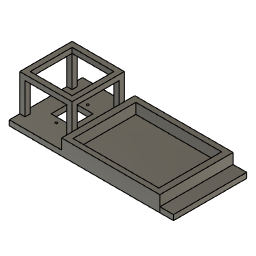
PDMS holder v6 (Autodesk Fusion 360 design; units mm, degrees)
Autodesk Fusion 360 part; units mm, degrees
sketch "Sketch1" plane through (0, 0, 0) normal (0, 0, 1) x (1, 0, 0)
  line L0 (12.5, -12.5) -> (-12.5, -12.5)
  line L1 (-12.5, -12.5) -> (-12.5, 12.5)
  line L2 (-12.5, 12.5) -> (12.5, 12.5)
  line L3 (12.5, 12.5) -> (12.5, -12.5)
  line L4 (12.5, -12.5) -> (-12.5, 12.5) construction
  line L5 (-12.5, -12.5) -> (12.5, 12.5) construction
  line L6 (10, -10) -> (-10, -10)
  line L7 (-10, -10) -> (-10, 10)
  line L8 (-10, 10) -> (10, 10)
  line L9 (10, 10) -> (10, -10)
  line L10 (10, -10) -> (-10, 10) construction
  line L11 (-10, -10) -> (10, 10) construction
  line L12 (5, -5) -> (-5, -5)
  line L13 (-5, -5) -> (-5, 5)
  line L14 (-5, 5) -> (5, 5)
  line L15 (5, 5) -> (5, -5)
  line L16 (5, -5) -> (-5, 5) construction
  line L17 (-5, -5) -> (5, 5) construction
  line L18 (12.5, 0) -> (12.5, 17.5)
  line L19 (12.5, 17.5) -> (59.5, 17.5)
  line L20 (59.5, 17.5) -> (59.5, -17.5)
  line L21 (59.5, -17.5) -> (12.5, -17.5)
  line L22 (12.5, -17.5) -> (12.5, 17.5)
  line L23 (12.5, 0) -> (36, 0)
  line L24 (56.5, -15) -> (15.5, -15)
  line L25 (15.5, -15) -> (15.5, 15)
  line L26 (15.5, 15) -> (56.5, 15)
  line L27 (56.5, 15) -> (56.5, -15)
  line L28 (56.5, -15) -> (15.5, 15) construction
  line L29 (15.5, -15) -> (56.5, 15) construction
  line L30 (12.5, -17.5) -> (-12.5, -17.5)
  line L31 (-12.5, -17.5) -> (-12.5, 17.5)
  line L32 (-12.5, 17.5) -> (12.5, 17.5)
  line L33 (12.5, 17.5) -> (12.5, -17.5)
  line L34 (0, 0) -> (0, 7.5)
  line L35 (0, 7.5) -> (0, -7.5)
  circle A0 centre (0, 7.5) radius 0.5
  circle A1 centre (0, -7.5) radius 0.5
  line L36 (59.5, 17.5) -> (66, 17.5)
  line L37 (66, 17.5) -> (66, -17.5)
  line L38 (66, -17.5) -> (59.5, -17.5)
  line L39 (59.5, -17.5) -> (59.5, 17.5)
  point P0 (36, 0)
  dimension "d1" = 25
  dimension "d2" = 25
  dimension "d3" = 20
  dimension "d4" = 20
  dimension "d19" = 10
  dimension "d20" = 10
  dimension "d25" = 17.5
  dimension "d26" = 47
  dimension "d27" = 35
  dimension "d28" = 23.5
  dimension "d29" = 41
  dimension "d30" = 30
  dimension "d33" = 25
  dimension "d34" = 35
  dimension "d35" = 7.5
  dimension "d36" = 15
  dimension "d37" = 1
  dimension "d38" = 1
  dimension "d39" = 6.5
  dimension "d40" = 35
  constraint horizontal L0
  constraint perpendicular L0 L1
  constraint parallel L0 L2
  constraint parallel L1 L3
  constraint coincident L4 L34.start
  constraint coincident L5 L34.start
  constraint coincident L34.start origin
  constraint horizontal L6
  constraint perpendicular L6 L7
  constraint parallel L6 L8
  constraint parallel L7 L9
  constraint coincident L10 L34.start
  constraint coincident L11 L34.start
  constraint horizontal L12
  constraint perpendicular L12 L13
  constraint parallel L12 L14
  constraint parallel L13 L15
  constraint coincident L16 L34.start
  constraint coincident L17 L34.start
  constraint midpoint L3 L18.start
  constraint perpendicular L2 L18
  constraint horizontal L19
  constraint vertical L20
  constraint horizontal L21
  constraint vertical L22
  constraint perpendicular L22 L23
  constraint horizontal L24
  constraint perpendicular L24 L25
  constraint parallel L24 L26
  constraint parallel L25 L27
  constraint coincident L28 P0
  constraint coincident L29 P0
  constraint coincident P0 L23.end
  constraint horizontal L30
  constraint vertical L31
  constraint horizontal L32
  constraint vertical L33
  constraint perpendicular L14 L34
  constraint parallel L34 L35
  constraint coincident L34.end L35.start
  constraint coincident L35.end A1.centre
  constraint horizontal L36
  constraint vertical L37
  constraint horizontal L38
  constraint vertical L39
  measures "d1" distance of L1.end L2.end
  measures "d2" distance of L0.end L1.end
  measures "d3" distance of L7.end L8.end
  measures "d4" distance of L6.end L7.end
  measures "d19" distance of L13.end L14.end
  measures "d20" distance of L12.end L13.end
  measures "d25" distance of L18.start L18.end
  measures "d26" distance of L18.end L19.end
  measures "d27" distance of L18.end L21.end
  measures "d28" distance of L18.start P0
  measures "d29" distance of L25.end L26.end
  measures "d30" distance of L24.end L25.end
  measures "d33" distance of L21.end L30.end
  measures "d34" distance of L21.end L18.end
  measures "d35" distance of L34.start L34.end
  measures "d36" distance of L34.end L35.end
  measures "d37" diameter of A0
  measures "d38" diameter of A1
  measures "d39" distance of L19.end L36.end
  measures "d40" distance of L19.end L20.end
extrude "Extrude1" add sketch "Sketch1" along normal blind 20 contours L0 L1 L2 L3 L18 L22 L31 L33 makes body 1
sketch "Sketch2" plane through (0, -12.5, 0) normal (0, -1, 0) x (1, 0, 0)
  line L0 (-12.5, 0) -> (12.5, 0)
  line L1 (12.5, 0) -> (12.5, 20)
  line L2 (12.5, 20) -> (-12.5, 20)
  line L3 (-12.5, 20) -> (-12.5, 0)
  line L4 (0, 0) -> (0, 10)
  line L5 (10, 2.5) -> (-10, 2.5)
  line L6 (-10, 2.5) -> (-10, 17.5)
  line L7 (-10, 17.5) -> (10, 17.5)
  line L8 (10, 17.5) -> (10, 2.5)
  line L9 (10, 2.5) -> (-10, 17.5) construction
  line L10 (-10, 2.5) -> (10, 17.5) construction
  point P0 (0, 10)
  dimension "d7" = 10
  dimension "d8" = 20
  dimension "d9" = 15
  constraint coincident L4.start origin
  constraint perpendicular L2 L4
  constraint horizontal L5
  constraint perpendicular L5 L6
  constraint parallel L5 L7
  constraint parallel L6 L8
  constraint coincident L9 P0
  constraint coincident L10 P0
  constraint coincident P0 L4.end
  measures "d7" distance of L4.start P0
  measures "d8" distance of L6.end L7.end
  measures "d9" distance of L5.end L6.end
extrude "Extrude2" cut sketch "Sketch2" against normal blind 25 contours L5 L6 L7 L8 bodies 1
sketch "Sketch3" plane through (12.5, 0, 0) normal (1, 0, 0) x (0, 1, 0)
  line L0 (-12.5, 0) -> (12.5, 0)
  line L1 (12.5, 0) -> (12.5, 20)
  line L2 (12.5, 20) -> (-12.5, 20)
  line L3 (-12.5, 20) -> (-12.5, 0)
  line L4 (0, 0) -> (0, 10)
  line L5 (10, 2.5) -> (-10, 2.5)
  line L6 (-10, 2.5) -> (-10, 17.5)
  line L7 (-10, 17.5) -> (10, 17.5)
  line L8 (10, 17.5) -> (10, 2.5)
  line L9 (10, 2.5) -> (-10, 17.5) construction
  line L10 (-10, 2.5) -> (10, 17.5) construction
  point P0 (0, 10)
  dimension "d12" = 10
  dimension "d13" = 20
  dimension "d14" = 15
  constraint vertical L4
  constraint coincident L4.start origin
  constraint horizontal L5
  constraint perpendicular L5 L6
  constraint parallel L5 L7
  constraint parallel L6 L8
  constraint coincident L9 P0
  constraint coincident L10 P0
  constraint coincident P0 L4.end
  measures "d12" distance of L4.start P0
  measures "d13" distance of L6.end L7.end
  measures "d14" distance of L5.end L6.end
extrude "Extrude3" cut sketch "Sketch3" against normal blind 25 contours L5 L6 L7 L8 bodies 1
extrude "Extrude4" add sketch "Sketch1" along normal blind 2.5 contours L0 L22 L30 L31 L33 | L2 L18 L22 L31 L32 L33 | L20 L36 L37 L38 L39 | L6 L7 L8 L9 | L24 L25 L26 L27 bodies 1 makes body 2 at (29.1667, -5, 0) makes body 3 at (61.6667, 5.8333, 0)
extrude "Extrude5" add sketch "Sketch1" along normal blind 7.5 contours L3 L18 L19 L20 L21 L22 L33 L39 bodies 1 2
